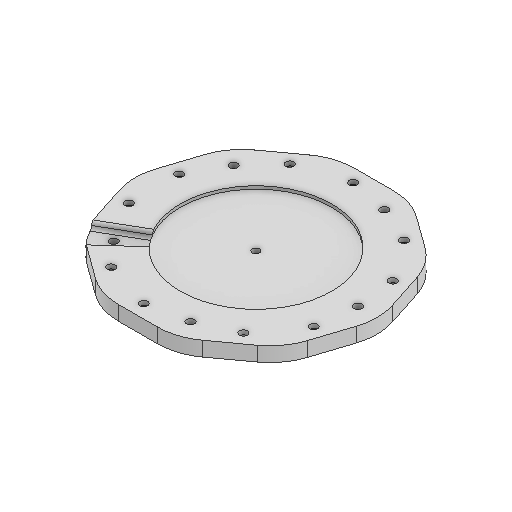
# Autodesk Inventor part: lidarCage
Saved by Autodesk Inventor 2025 (Build 290162000, 162)
## iProperties
Created: 2024-12-07
Part Number: lidarCage
Material: Generic
Document SubType Name: Modeling
Designer: derm
Density: 1 g/cm^3
Appearance: Default
Author: derm
Autodesk Inventor part; units mm, degrees
ref_plane "YZ Plane" through (0, 0, 0) normal (1, 0, 0) x (0, 1, 0)
ref_plane "XZ Plane" through (0, 0, 0) normal (0, 1, 0) x (-1, 0, 0)
ref_plane "XY Plane" through (0, 0, 0) normal (0, 0, 1) x (1, 0, 0)
sketch "Sketch1" plane through (0, 0, 0) normal (0, 1, 0) x (-1, 0, 0)
  circle A0 centre (0, 0) radius 52
  circle A1 centre (0, 0) radius 2.5
  dimension "d0" = 104
  dimension "d1" = 5
  constraints: 2 centre point, 2 coincident
  measures "d0" diameter of A0
  measures "d1" diameter of A1
extrude "Extrusion1" add sketch "Sketch1" along normal blind 8
sketch "Sketch2" plane through (0, 0, 0) normal (0, -1, 0) x (1, 0, 0)
  circle A0 centre (0, 0) radius 52 projected
  circle A1 centre (0, 0) radius 2.5 projected
  line L0 (85.2574, 0) -> (68.9747, -50.113)
  line L1 (68.9747, -50.113) -> (26.346, -81.0846)
  line L2 (26.346, -81.0846) -> (-26.346, -81.0846)
  line L3 (-26.346, -81.0846) -> (-68.9747, -50.113)
  line L4 (-68.9747, -50.113) -> (-85.2574, 0)
  line L5 (-85.2574, 0) -> (-68.9747, 50.113)
  line L6 (-68.9747, 50.113) -> (-26.346, 81.0846)
  line L7 (-26.346, 81.0846) -> (26.346, 81.0846)
  line L8 (26.346, 81.0846) -> (68.9747, 50.113)
  line L9 (68.9747, 50.113) -> (85.2574, 0)
  constraints: 20 end point, 1 coincident, 21 other
extrude "Extrusion2" add sketch "Sketch2" against normal blind 10 contours L0 L1 L2 L3 L4 L5 L6 L7 L8 L9
sketch "Sketch3" plane through (0, 0, 0) normal (0, -1, 0) x (1, 0, 0)
  line L0 (68.9747, 50.113) -> (26.346, 81.0846) projected
  line L1 (26.346, 81.0846) -> (-26.346, 81.0846) projected
  line L2 (-26.346, 81.0846) -> (-68.9747, 50.113) projected
  line L3 (-68.9747, 50.113) -> (-85.2574, 0) projected
  line L4 (-85.2574, 0) -> (-68.9747, -50.113) projected
  line L5 (-68.9747, -50.113) -> (-26.346, -81.0846) projected
  line L6 (-26.346, -81.0846) -> (26.346, -81.0846) projected
  line L7 (26.346, -81.0846) -> (68.9747, -50.113) projected
  line L8 (68.9747, -50.113) -> (85.2574, 0) projected
  line L9 (85.2574, 0) -> (68.9747, 50.113) projected
  circle A0 centre (0, 0) radius 2.5 projected
  line L10 (-19.05, 69.85) -> (19.05, 69.85) construction
  line L11 (-19.05, 67.1) -> (19.05, 67.1)
  line L12 (19.05, 72.6) -> (-19.05, 72.6)
  arc A1 (-19.05, 72.6) -> (-19.05, 67.1) centre (-19.05, 69.85) ccw
  arc A2 (19.05, 67.1) -> (19.05, 72.6) centre (19.05, 69.85) ccw
  arc A3 (-48.5853, 50.0478) -> (-53.3484, 52.7978) centre (-50.9669, 51.4228) ccw
  line L13 (-67.6353, 17.0522) -> (-48.5853, 50.0478)
  line L14 (-53.3484, 52.7978) -> (-72.3984, 19.8022)
  arc A4 (-72.3984, 19.8022) -> (-67.6353, 17.0522) centre (-70.0169, 18.4272) ccw
  line L15 (-70.0169, 18.4272) -> (-50.9669, 51.4228) construction
  arc A5 (-67.6353, -17.0522) -> (-72.3984, -19.8022) centre (-70.0169, -18.4272) ccw
  line L16 (-48.5853, -50.0478) -> (-67.6353, -17.0522)
  line L17 (-72.3984, -19.8022) -> (-53.3484, -52.7978)
  arc A6 (-53.3484, -52.7978) -> (-48.5853, -50.0478) centre (-50.9669, -51.4228) ccw
  line L18 (-50.9669, -51.4228) -> (-70.0169, -18.4272) construction
  arc A7 (-19.05, -67.1) -> (-19.05, -72.6) centre (-19.05, -69.85) ccw
  line L19 (19.05, -67.1) -> (-19.05, -67.1)
  line L20 (-19.05, -72.6) -> (19.05, -72.6)
  arc A8 (19.05, -72.6) -> (19.05, -67.1) centre (19.05, -69.85) ccw
  line L21 (19.05, -69.85) -> (-19.05, -69.85) construction
  arc A9 (48.5853, -50.0478) -> (53.3484, -52.7978) centre (50.9669, -51.4228) ccw
  line L22 (67.6353, -17.0522) -> (48.5853, -50.0478)
  line L23 (53.3484, -52.7978) -> (72.3984, -19.8022)
  arc A10 (72.3984, -19.8022) -> (67.6353, -17.0522) centre (70.0169, -18.4272) ccw
  line L24 (70.0169, -18.4272) -> (50.9669, -51.4228) construction
  arc A11 (67.6353, 17.0522) -> (72.3984, 19.8022) centre (70.0169, 18.4272) ccw
  line L25 (48.5853, 50.0478) -> (67.6353, 17.0522)
  line L26 (72.3984, 19.8022) -> (53.3484, 52.7978)
  arc A12 (53.3484, 52.7978) -> (48.5853, 50.0478) centre (50.9669, 51.4228) ccw
  line L27 (50.9669, 51.4228) -> (70.0169, 18.4272) construction
  point P0 (0, 69.85)
  point P1 (-60.4919, 34.925)
  point P2 (-60.4919, -34.925)
  point P3 (0, -69.85)
  point P4 (60.4919, -34.925)
  point P5 (60.4919, 34.925)
  dimension "d6" = 38.1
  dimension "d7" = 69.85
  dimension "d8" = 2.75
  dimension "d11" = 360
  constraints: 48 end point, 24 point on circle, 12 centre point, 4 tangent, 1 horizontal, 1 midpoint, 1 parallel, 73 other
  measures "d6" distance of L10.start L10.end
  measures "d7" distance of point (0, 0) point (0, 69.85)
  measures "d8" radius of A1
sketch "Sketch4" plane through (0, 10, 0) normal (0, 1, 0) x (1, 0, 0)
  line L0 (68.9747, -50.113) -> (85.2574, 0) projected
  line L1 (85.2574, 0) -> (68.9747, 50.113) projected
  line L2 (68.9747, 50.113) -> (26.346, 81.0846) projected
  line L3 (26.346, 81.0846) -> (-26.346, 81.0846) projected
  line L4 (-26.346, 81.0846) -> (-68.9747, 50.113) projected
  line L5 (-68.9747, 50.113) -> (-85.2574, 0) projected
  line L6 (-85.2574, 0) -> (-68.9747, -50.113) projected
  line L7 (-68.9747, -50.113) -> (-26.346, -81.0846) projected
  line L8 (-26.346, -81.0846) -> (26.346, -81.0846) projected
  line L9 (26.346, -81.0846) -> (68.9747, -50.113) projected
  circle A0 centre (0, 0) radius 52 projected
  circle A1 centre (0, 0) radius 2.5 projected
  line L10 (0, 0) -> (-71.7901, -41.448)
  line L11 (0, 0) -> (-61.6038, -55.4683)
  line L12 (-68.9747, -50.113) -> (0, 0)
  arc A2 (-13.8064, -0.992) -> (-13.6688, 2.1578) centre (-13.7376, 0.5829) ccw projected
  line L13 (-13.8064, -0.992) -> (-43.7214, 0.3141) projected
  arc A3 (-43.5839, 3.4639) -> (-43.7214, 0.3141) centre (-43.6527, 1.889) ccw projected
  line L14 (-43.5839, 3.4639) -> (-13.6688, 2.1578) projected
  arc A4 (-11.7527, 7.3126) -> (-9.79, 9.78) centre (-10.7714, 8.5463) ccw projected
  line L15 (-11.7527, 7.3126) -> (-35.1867, 25.9529) projected
  arc A5 (-33.2241, 28.4203) -> (-35.1867, 25.9529) centre (-34.2054, 27.1866) ccw projected
  line L16 (-33.2241, 28.4203) -> (-9.79, 9.78) projected
  arc A6 (-5.2099, 12.8241) -> (-2.1717, 13.6666) centre (-3.6908, 13.2454) ccw projected
  line L17 (-5.2099, 12.8241) -> (-13.2119, 41.6786) projected
  arc A7 (-10.1738, 42.5211) -> (-13.2119, 41.6786) centre (-11.6929, 42.0999) ccw projected
  line L18 (-10.1738, 42.5211) -> (-2.1717, 13.6666) projected
  arc A8 (3.3229, 13.4372) -> (6.2761, 12.3331) centre (4.7995, 12.8851) ccw projected
  line L19 (3.3229, 13.4372) -> (13.8094, 41.4845) projected
  arc A9 (16.7625, 40.3803) -> (13.8094, 41.4845) centre (15.286, 40.9324) ccw projected
  line L20 (16.7625, 40.3803) -> (6.2761, 12.3331) projected
  arc A10 (10.5865, 8.9177) -> (12.3266, 6.2887) centre (11.4566, 7.6032) ccw projected
  line L21 (10.5865, 8.9177) -> (35.556, 25.4447) projected
  arc A11 (37.2961, 22.8156) -> (35.556, 25.4447) centre (36.4261, 24.1302) ccw projected
  line L22 (37.2961, 22.8156) -> (12.3266, 6.2887) projected
  arc A12 (13.8064, 0.992) -> (13.6688, -2.1578) centre (13.7376, -0.5829) ccw projected
  line L23 (13.8064, 0.992) -> (43.7214, -0.3141) projected
  arc A13 (43.5839, -3.4639) -> (43.7214, -0.3141) centre (43.6527, -1.889) ccw projected
  line L24 (43.5839, -3.4639) -> (13.6688, -2.1578) projected
  arc A14 (11.7527, -7.3126) -> (9.79, -9.78) centre (10.7714, -8.5463) ccw projected
  line L25 (11.7527, -7.3126) -> (35.1867, -25.9529) projected
  arc A15 (33.2241, -28.4203) -> (35.1867, -25.9529) centre (34.2054, -27.1866) ccw projected
  line L26 (33.2241, -28.4203) -> (9.79, -9.78) projected
  arc A16 (5.2099, -12.8241) -> (2.1717, -13.6666) centre (3.6908, -13.2454) ccw projected
  line L27 (5.2099, -12.8241) -> (13.2119, -41.6786) projected
  arc A17 (10.1738, -42.5211) -> (13.2119, -41.6786) centre (11.6929, -42.0999) ccw projected
  line L28 (10.1738, -42.5211) -> (2.1717, -13.6666) projected
  arc A18 (-3.3229, -13.4372) -> (-6.2761, -12.3331) centre (-4.7995, -12.8851) ccw projected
  line L29 (-3.3229, -13.4372) -> (-13.8094, -41.4845) projected
  arc A19 (-16.7625, -40.3803) -> (-13.8094, -41.4845) centre (-15.286, -40.9324) ccw projected
  line L30 (-16.7625, -40.3803) -> (-6.2761, -12.3331) projected
  arc A20 (-10.5865, -8.9177) -> (-12.3266, -6.2887) centre (-11.4566, -7.6032) ccw projected
  line L31 (-10.5865, -8.9177) -> (-35.556, -25.4447) projected
  arc A21 (-37.2961, -22.8156) -> (-35.556, -25.4447) centre (-36.4261, -24.1302) ccw projected
  line L32 (-37.2961, -22.8156) -> (-12.3266, -6.2887) projected
  point P0 (-45.0333, -26)
  point P1 (-38.6435, -34.7948)
  dimension "d13" = 6
  dimension "d14" = 6
  constraints: 6 end point, 2 point on line
  measures "d13" angle of L12 L11
  measures "d14" angle of L12 L10
extrude "Extrusion3" cut sketch "Sketch4" against normal blind 4 contours L7 L12 A0 L11 | L6 L10 A0 L12
fillet "Fillet1" radius 2 4 edges at (-50.1237, 6, 45.1315) (-50.1237, 10, 45.1315) (-58.4117, 6, 33.724) (-58.4117, 10, 33.724)
sketch "Sketch5" plane through (0, 0, 0) normal (0, -1, 0) x (1, 0, 0)
  circle A0 centre (0, 0) radius 2.5 projected
  circle A1 centre (0, 0) radius 4.25
  dimension "d18" = 8.5
  constraints: 1 centre point, 1 coincident
  measures "d18" diameter of A1
extrude "Extrusion4" cut sketch "Sketch5" against normal blind 4
sketch "Sketch6" plane through (0, 10, 0) normal (0, 1, 0) x (1, 0, 0)
  circle A0 centre (-5.2226, 71.9683) radius 2.75 projected
  circle A1 centre (-38.0767, 61.2934) radius 2.75 projected
  point P0 (0, 0)
extrude "Extrusion5" cut sketch "Sketch6" against normal through all
sketch "Sketch7" plane through (0, 0, 0) normal (0, -1, 0) x (1, 0, 0)
  circle A0 centre (-5.2226, -71.9683) radius 2.75 projected
  circle A1 centre (-38.0767, -61.2934) radius 2.75 projected
  line L0 (-3.2088, -76.1249) -> (-7.8155, -75.7906)
  line L1 (-7.8155, -75.7906) -> (-9.8293, -71.634)
  line L2 (-9.8293, -71.634) -> (-7.2365, -67.8116)
  line L3 (-7.2365, -67.8116) -> (-2.6298, -68.1459)
  line L4 (-2.6298, -68.1459) -> (-0.6159, -72.3026)
  line L5 (-0.6159, -72.3026) -> (-3.2088, -76.1249)
  circle A2 centre (-38.0767, -61.2934) radius 2.75 projected
  line L6 (-42.1783, -63.4171) -> (-41.9667, -58.8031)
  line L7 (-41.9667, -58.8031) -> (-37.8651, -56.6794)
  line L8 (-37.8651, -56.6794) -> (-33.9751, -59.1696)
  line L9 (-33.9751, -59.1696) -> (-34.1867, -63.7836)
  line L10 (-34.1867, -63.7836) -> (-38.2883, -65.9073)
  line L11 (-38.2883, -65.9073) -> (-42.1783, -63.4171)
  circle A3 centre (0, 0) radius 4.25 projected
  line L12 (-5.2226, -71.9683) -> (0, 0) construction
  circle A4 centre (0, 0) radius 2.5 projected
  line L13 (-38.0767, -61.2934) -> (0, 0) construction
  point P0 (-4.9331, -67.9788)
  dimension "d23" = 8
  dimension "d24" = 8
  constraints: 28 end point, 2 coincident, 1 midpoint, 1 point on line, 26 other
  measures "d23" distance from line of point (-4.933, -67.979) L0
  measures "d24" distance between parallel lines of L8 L11
extrude "Extrusion6" cut sketch "Sketch7" against normal blind 7 contours L0 L1 L2 L3 L4 L5 | L6 L7 L8 L9 L10 L11
pattern_circular "Circular Pattern1" count 5 over 360 about axis through (0, -10, 0) along (0, 1, 0) of "Extrusion6", "Extrusion5"
fillet "Fillet2" radius 40 10 edges at (-68.9747, 5, -50.113) (-85.2574, 5, 0) (-26.346, 5, -81.0846) (26.346, 5, -81.0846) (68.9747, 5, -50.113) (85.2574, 5, 0) (68.9747, 5, 50.113) (26.346, 5, 81.0846) (-26.346, 5, 81.0846) (-68.9747, 3, 50.113)
sketch "Sketch8" plane through (0, 10, 0) normal (0, 1, 0) x (1, 0, 0)
  arc A0 (-11.7527, 7.3126) -> (-9.79, 9.78) centre (-10.7714, 8.5463) ccw projected
  line L0 (-11.7527, 7.3126) -> (-35.1867, 25.9529) projected
  arc A1 (-33.2241, 28.4203) -> (-35.1867, 25.9529) centre (-34.2054, 27.1866) ccw projected
  line L1 (-33.2241, 28.4203) -> (-9.79, 9.78) projected
  arc A2 (3.3229, 13.4372) -> (6.2761, 12.3331) centre (4.7995, 12.8851) ccw projected
  line L2 (3.3229, 13.4372) -> (13.8094, 41.4845) projected
  arc A3 (16.7625, 40.3803) -> (13.8094, 41.4845) centre (15.286, 40.9324) ccw projected
  line L3 (16.7625, 40.3803) -> (6.2761, 12.3331) projected
  arc A4 (13.8064, 0.992) -> (13.6688, -2.1578) centre (13.7376, -0.5829) ccw projected
  line L4 (13.8064, 0.992) -> (43.7214, -0.3141) projected
  arc A5 (43.5839, -3.4639) -> (43.7214, -0.3141) centre (43.6527, -1.889) ccw projected
  line L5 (43.5839, -3.4639) -> (13.6688, -2.1578) projected
  arc A6 (5.2099, -12.8241) -> (2.1717, -13.6666) centre (3.6908, -13.2454) ccw projected
  line L6 (5.2099, -12.8241) -> (13.2119, -41.6786) projected
  arc A7 (10.1738, -42.5211) -> (13.2119, -41.6786) centre (11.6929, -42.0999) ccw projected
  line L7 (10.1738, -42.5211) -> (2.1717, -13.6666) projected
  arc A8 (-10.5865, -8.9177) -> (-12.3266, -6.2887) centre (-11.4566, -7.6032) ccw projected
  line L8 (-10.5865, -8.9177) -> (-35.556, -25.4447) projected
  arc A9 (-37.2961, -22.8156) -> (-35.556, -25.4447) centre (-36.4261, -24.1302) ccw projected
  line L9 (-37.2961, -22.8156) -> (-12.3266, -6.2887) projected
  arc A10 (36.8606, 73.4453) -> (13.3492, 81.0846) centre (13.3492, 41.0846) ccw projected
  line L10 (13.3492, 81.0846) -> (-13.3492, 81.0846) projected
  arc A11 (-13.3492, 81.0846) -> (-36.8606, 73.4453) centre (-13.3492, 41.0846) ccw projected
  line L11 (-36.8606, 73.4453) -> (-58.46, 57.7524) projected
  arc A12 (-58.46, 57.7524) -> (-72.9909, 37.7524) centre (-34.9486, 25.3917) ccw projected
  line L12 (-72.9909, 37.7524) -> (-81.2412, 12.3607) projected
  arc A13 (-81.2412, 12.3607) -> (-81.2412, -12.3607) centre (-43.1989, 0) ccw projected
  line L13 (-81.2412, -12.3607) -> (-72.9909, -37.7524) projected
  arc A14 (-72.9909, -37.7524) -> (-58.46, -57.7524) centre (-34.9486, -25.3917) ccw projected
  line L14 (-58.46, -57.7524) -> (-36.8606, -73.4453) projected
  arc A15 (-36.8606, -73.4453) -> (-13.3492, -81.0846) centre (-13.3492, -41.0846) ccw projected
  line L15 (-13.3492, -81.0846) -> (13.3492, -81.0846) projected
  arc A16 (13.3492, -81.0846) -> (36.8606, -73.4453) centre (13.3492, -41.0846) ccw projected
  line L16 (36.8606, -73.4453) -> (58.46, -57.7524) projected
  arc A17 (58.46, -57.7524) -> (72.9909, -37.7524) centre (34.9486, -25.3917) ccw projected
  line L17 (72.9909, -37.7524) -> (81.2412, -12.3607) projected
  arc A18 (81.2412, -12.3607) -> (81.2412, 12.3607) centre (43.1989, 0) ccw projected
  line L18 (81.2412, 12.3607) -> (72.9909, 37.7524) projected
  arc A19 (72.9909, 37.7524) -> (58.46, 57.7524) centre (34.9486, 25.3917) ccw projected
  line L19 (58.46, 57.7524) -> (36.8606, 73.4453) projected
  circle A20 centre (70, 0) radius 2.75
  point P0 (0, 0)
  dimension "d31" = 70
  dimension "d32" = 5.5
  constraints: 1 centre point
  measures "d31" distance of A20.centre point (0, 0)
  measures "d32" diameter of A20
extrude "Extrusion7" cut sketch "Sketch8" against normal through all contours A20
pattern_circular "Circular Pattern2" count 5 over 360 about axis through (0, -10, 0) along (0, 1, 0) of "Extrusion7"
body "Solid1"
